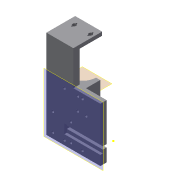
# Autodesk Inventor part: cellSTORM_inverted_Laser_10x_laserscanner_left_v2
Saved by Autodesk Inventor 2019.4 (Build 234330000, 330)
## iProperties
Created: 2020-11-05
Part Number: cellSTORM_inverted_Laser_10x_laserscanner_left_v2
Material: Generic
Document SubType Name: Modeling
Designer: diederichbenedict
Density: 1 g/cm^3
Appearance: Default
Author: diederichbenedict
Autodesk Inventor part; units mm, degrees
ref_plane "YZ Plane" through (0, 0, 0) normal (1, 0, 0) x (0, 1, 0)
ref_plane "Work Plane16" through (-37.5, 5.5, 41.5) normal (0, 0, -1) x (-1, 0, 0)
sketch "Sketch19" plane through (-37.5, 5.5, 41.5) normal (0, 0, -1) x (-1, 0, 0)
  circle A0 centre (-10, -25) radius 1.45 construction
  circle A1 centre (10, -25) radius 1.45 construction
  circle A2 centre (10, 25) radius 1.45 construction
  line L0 (-30, 28) -> (-30, -28) construction
  line L1 (28, 30) -> (-28, 30) construction
  line L2 (-30, -28) -> (-30, 28) construction
  line L3 (30, 28) -> (30, -28) construction
  line L4 (-28, -30) -> (28, -30) construction
  line L5 (-30, 0) -> (12.4264, 0) construction
  line L6 (0, 30) -> (30, 30)
  line L7 (30, 30) -> (30, 0)
  line L8 (30, 0) -> (41.9908, 0)
  line L9 (41.9908, -33.8566) -> (30, -30)
  line L10 (30, -30) -> (-30, -30)
  line L11 (-30, -30) -> (-30, 0)
  circle A3 centre (10, -25) radius 1.45
  circle A4 centre (10, 25) radius 1.45
  line L12 (0.5, 63.5) -> (25.5, 63.5)
  line L13 (0.5, 64.5) -> (25.5, 64.5)
  line L14 (30, 30) -> (0, 30)
  line L15 (0, 30) -> (0, 68.5)
  line L16 (0, 68.5) -> (30, 68.5)
  line L17 (30, 68.5) -> (30, 30)
  line L18 (0, 30) -> (-30, 30)
  line L19 (-30, 30) -> (-30, 0)
  circle A5 centre (-10, 25) radius 1.5209
  line L20 (30, 0.4817) -> (30, -30)
  circle A6 centre (-10, -25) radius 1.45
  point P0 (-37.5, -5.5)
  dimension "d106" = 4
  constraints: 42 end point, 8 horizontal, 7 centre point, 3 coincident, 3 concentric, 3 midpoint, 3 parallel, 3 vertical, 2 point on line, 1 collinear, 1 perpendicular, 18 other
  measures "d106" distance between parallel lines of L13 L16
extrude "Extrusion16" add sketch "Sketch19" along normal blind 7
ref_plane "Work Plane18" through (-80.5, 4.5, 11.5376) normal (0, 1, 0) x (0, 0, 1)
ref_plane "Work Plane19" through (-100.5, 11.5, 5.5) normal (0, 1, 0) x (0, 0, 1)
sketch "Sketch20" plane through (-79.4908, -24.5, 41.5) normal (0, 1, 0) x (1, 0, 0)
  line L0 (11.9908, 7) -> (41.9908, 7) projected
  line L1 (-5.0092, 36) -> (4.7181, 36)
  line L2 (4.7181, 36) -> (4.7181, 15.0376)
  line L3 (4.7181, 15.0376) -> (-5.0092, 15.0376)
  line L4 (21.7615, 7) -> (4.7181, 36)
  line L5 (21.7615, 7) -> (11.9908, 7)
  line L6 (-5.0092, 20.603) -> (-5.0092, 32.1376)
  line L7 (-5.0092, 36) -> (-5.0092, 15.0376)
  line L8 (-6.0092, 36) -> (-5.0092, 36)
  line L9 (-6.0092, 15.0376) -> (-5.0092, 15.0376)
  line L10 (4.7181, 15.0376) -> (11.9908, 15.0376)
  line L11 (11.9908, 15.0376) -> (11.9908, 7)
  point P0 (79.4908, 41.5)
  point P1 (28.1756, 7)
  dimension "d161" = 0
  dimension "d162" = 0
  constraints: 22 end point, 4 horizontal, 3 perpendicular, 1 collinear, 1 parallel, 1 point on line, 1 vertical, 6 other
  measures "d161" distance between parallel lines of L8 L1
  measures "d162" distance between parallel lines of L9 L3
extrude "Extrusion17" add sketch "Sketch20" along normal up to surface (36 mm away)
sketch "Sketch21" plane through (-84.5, -28.3595, 5.5) normal (-1, 0, 0) x (0, 0, 1)
  circle A0 centre (17.7, 9.3595) radius 1
  circle A1 centre (2.2, 30.8595) radius 1
  circle A2 centre (22.7, 37.3595) radius 1
  circle A3 centre (12.7, 19.8595) radius 2.6486
  line L0 (6.3352, 35.6445) -> (19.7051, 35.6445)
  line L1 (19.7051, 35.6445) -> (19.7051, 12.3611)
  line L2 (19.7051, 12.3611) -> (6.3352, 12.3611)
  line L3 (6.3352, 12.3611) -> (6.3352, 35.6445)
  line L4 (6.3352, 35.6445) -> (19.7051, 12.3611) construction
  line L5 (19.7051, 35.6445) -> (6.3352, 12.3611) construction
  circle A4 centre (17.7, 9.3595) radius 0.75
  circle A5 centre (2.2, 30.8595) radius 0.75
  circle A6 centre (22.7, 37.3595) radius 0.75
  point P0 (13.0201, 24.0028)
  dimension "d154" = 1.5
  dimension "d155" = 1.5
  dimension "d156" = 1.5
  constraints: 12 end point, 7 centre point, 3 coincident, 2 midpoint, 2 parallel, 1 horizontal, 1 perpendicular, 8 other
  measures "d154" diameter of A4
  measures "d155" diameter of A5
  measures "d156" diameter of A6
extrude "Extrusion18" cut sketch "Sketch21" against normal through all contours A3 | L0 L1 L2 L3 | A4 | A5 | A6
sketch "Sketch23" plane through (-37.5, 5.5, 34.5) normal (0, 0, -1) x (-1, 0, 0)
  line L0 (30, 6) -> (30, 68.5) projected
  line L1 (30, 68.5) -> (0, 68.5) projected
  line L2 (0, 68.5) -> (0, 30) projected
  line L3 (-30, 30) -> (-30, -30) projected
  line L4 (-30, -30) -> (20.2293, -30) projected
  circle A0 centre (10, -25) radius 1.45 projected
  circle A1 centre (10, 25) radius 1.45 projected
  line L5 (30, 68.5) -> (0, 68.5) projected
  line L6 (0.5, 64.5) -> (25.5, 64.5)
  line L7 (30, 68.5) -> (0, 68.5)
  line L8 (0, 68.5) -> (0, 64.5)
  line L9 (0, 64.5) -> (30, 64.5)
  line L10 (30, 64.5) -> (30, 68.5)
  line L11 (0, 30) -> (-30, 30) projected
  line L12 (20.2293, 6) -> (30, 6) projected
  line L13 (20.2293, -30) -> (20.2293, 6) projected
  point P0 (-37.5, -5.5)
  constraints: 10 end point, 2 horizontal, 2 parallel, 1 perpendicular, 1 point on line, 2 other
extrude "Extrusion20" add sketch "Sketch23" along normal blind 25 contours L9 L6 L2 L1 L0
sketch "Sketch24" plane through (-67.5, 74, 41.5) normal (0, 1, 0) x (1, 0, 0)
  circle A0 centre (6.5, 16.125) radius 1
  arc A1 (26, 21) -> (26, 25) centre (26, 23) ccw
  arc A2 (8, 25) -> (8, 21) centre (8, 23) ccw
  point P0 (67.5, 41.5)
  constraints: 4 point on circle, 3 centre point, 10 other
hole "Hole4" at (-59.5, 74, 18.5) at (-41.5, 74, 18.5) direction (0, -1, 0) diameter 4 depth 20 tip angle 118
sketch "Sketch25" plane through (-7.5, -24.5, 41.5) normal (1, 0, 0) x (0, 0, -1)
  line L0 (8, 17.4) -> (13.6, 17.4)
  line L1 (8, 14.6) -> (13.6, 14.6)
  line L2 (0, 0) -> (0, 98.5) projected
  line L3 (0, 21.0329) -> (2.8171, 21.0329)
  line L4 (2.8171, 21.0329) -> (2.8171, 10.7174)
  line L5 (2.8171, 10.7174) -> (0, 10.7174)
  line L6 (0, 10.7174) -> (0, 21.0329)
  line L7 (0.911, 17.6) -> (8.1191, 17.6)
  line L8 (8.1191, 17.6) -> (8.1191, 14.4)
  line L9 (8.1191, 14.4) -> (0.911, 14.4)
  line L10 (0.911, 14.4) -> (0.911, 17.6)
  line L11 (0.911, 17.6) -> (8.1191, 14.4) construction
  line L12 (8.1191, 17.6) -> (0.911, 14.4) construction
  circle A0 centre (23, 16) radius 2.5
  point P0 (41.5, 24.5)
  point P1 (4.5151, 16)
  dimension "d116" = 3.2
  dimension "d117" = 0
  constraints: 24 end point, 4 horizontal, 4 parallel, 2 midpoint, 2 perpendicular, 1 centre point, 1 point on line, 6 other
  measures "d116" distance of L7.end L8.end
  measures "d117" vertical distance of point (4.515, 16) A0.centre
extrude "Extrusion21" cut sketch "Sketch25" against normal blind 40 contours L2 L3 L4 L7 L10 L9 L5 | L9 L10 L7 L4 | L4 L7 L8 L9
ref_plane "Work Plane17" through (-65.74, 21.754, 18.5) normal (0, 1, 0) x (1, 0, 0)
sketch "Sketch26" plane through (-65.74, 21.754, 18.5) normal (0, 1, 0) x (1, 0, 0)
  circle A0 centre (15.24, 0) radius 15.24
  circle A1 centre (15.24, 0) radius 15.44
  line L0 (30.6779, -0.2548) -> (35.3241, -0.2548)
  line L1 (35.3241, -0.2548) -> (35.3241, -16)
  line L2 (58.24, -16) -> (8.0107, -16) projected
  line L3 (1.3147, -16) -> (35.3241, -16)
  arc A2 (-0.1726, -0.9196) -> (30.6779, -0.2548) centre (15.24, 0) ccw
  line L4 (-1.76, -16) -> (-1.76, -0.2548)
  line L5 (-1.76, -0.2548) -> (-0.1979, -0.2548)
  line L6 (-1.76, -16) -> (28.24, -16) projected
  line L7 (-1.76, -16) -> (28.24, -16)
  point P0 (65.74, 18.5)
  point P1 (14.4247, -16)
  dimension "d120" = 0.2
  constraints: 12 end point, 5 point on circle, 3 centre point, 3 horizontal, 2 concentric, 2 perpendicular, 1 point on line, 1 vertical, 2 other
  measures "d120" radial gap between concentric circles of A0 A1
extrude "Extrusion22" add sketch "Sketch26" along normal up to surface (24 mm away) from surface at -10.254 contours A1 L0 L1 L2 L3 L6 L4 L5
sketch "Sketch27" plane through (-30.4159, 35.5, 18.7548) normal (0, 0, -1) x (1, 0, 0)
  line L0 (-4.6462, 0) -> (0, 0) projected
  line L1 (-4.6462, 24) -> (-4.6462, 0) projected
  line L2 (0, 24) -> (0, 0) projected
  line L3 (-4.6462, 24) -> (0, 24) projected
  point P0 (30.4159, 35.5)
  point P1 (-2.3667, 19.6692)
  point P2 (-2.1061, 5.0728)
  point P3 (-54.438, 29.3311)
  point P4 (-55.6864, 54.2345)
  point P5 (7.1017, 19.6692)
hole "Hole5" at (-32.7825, 15.8308, 18.7548) at (-32.522, 30.4272, 18.7548) at (-86.1023, -18.7345, 18.7548) at (-84.8539, 6.1689, 18.7548) at (-23.3142, 15.8308, 18.7548) direction (0, 0, 1) diameter 2.9 end through all both
sketch "Sketch28" plane through (-37.5, 5.5, 34.5) normal (0, 0, -1) x (-1, 0, 0)
  point P0 (-37.5, -5.5)
sketch "Sketch29" plane through (-37.5, 5.5, 34.5) normal (0, 0, -1) x (-1, 0, 0)
  circle A0 centre (10, -25) radius 1.45 projected
  line L0 (-30, 30) -> (-30, -12.4) projected
  line L1 (-30, -12.4) -> (10, -12.4) projected
  line L2 (10, -12.4) -> (10, -15.6) projected
  line L3 (10, -15.6) -> (-30, -15.6) projected
  line L4 (-30, -15.6) -> (-30, -30) projected
  line L5 (-30, -30) -> (20.2293, -30) projected
  line L6 (12, -13) -> (13, -14)
  line L7 (4.9159, -8.7443) -> (17.0576, -20.886)
  line L8 (17.0576, -20.886) -> (14.9363, -23.0073)
  line L9 (14.9363, -23.0073) -> (2.7946, -10.8656)
  line L10 (2.7946, -10.8656) -> (4.9159, -8.7443)
  line L11 (6.3301, -7.3301) -> (18.4718, -19.4718)
  line L12 (18.4718, -19.4718) -> (20.5931, -17.3505)
  line L13 (20.5931, -17.3505) -> (8.4514, -5.2088)
  line L14 (8.4514, -5.2088) -> (6.3301, -7.3301)
  line L15 (30, 6) -> (30, 64.5) projected
  line L16 (30, 64.5) -> (0, 64.5) projected
  line L17 (0, 64.5) -> (0, 30) projected
  line L18 (0, 30) -> (-30, 30) projected
  line L19 (20.2293, -30) -> (20.2293, 6) projected
  line L20 (20.2293, 6) -> (30, 6) projected
  point P0 (-37.5, -5.5)
  dimension "d132" = 3
  dimension "d133" = 3
  dimension "d134" = 0
  dimension "d135" = 0
  dimension "d136" = 2
  dimension "d137" = 0
  constraints: 18 end point, 4 parallel, 2 perpendicular, 3 other
  measures "d132" distance between parallel lines of L7 L9
  measures "d133" distance between parallel lines of L13 L11
  measures "d134" distance between parallel lines of L14 L10
  measures "d135" distance between parallel lines of L12 L8
  measures "d136" distance between parallel lines of L11 L7
  measures "d137" distance between parallel lines of L11 L6
extrude "Extrusion23" add sketch "Sketch29" along normal blind 10 contours L9 L10 L7 L1 | L1 L7 L2 L3 L9 | L3 L2 L7 L8 L9 | L19 L12 L11 L6 L14 L13 | L13 L12 L19
sketch "Sketch30" plane through (-52.4363, -17.5073, 34.5) normal (0.7071068, -0.7071068, 0) x (-0.7071068, -0.7071068, 0)
  line L0 (0, 0) -> (-10.4755, 0) projected
  line L1 (0, 0) -> (0, 10) projected
  line L2 (-17.1709, 10) -> (0, 10) projected
  line L3 (-17.1709, 0) -> (-17.1709, 10) projected
  line L4 (-15.001, 0) -> (-17.1709, 0) projected
  line L5 (-10.4755, 0) -> (-15.001, 0) projected
  ellipse E0 centre (-38.851, 16) end of major axis (-38.851, 0.56) minor radius 10.9177 (-49.7672, 15.7452) -> (-27.9347, 15.7452) ccw projected
  circle A0 centre (-29.7987, 7.3684) radius 1.45
  circle A1 centre (-13.6778, 7.3684) radius 1.45
  circle A2 centre (-3.6035, 7.3684) radius 1.45
  point P0 (-49.4576, 34.5)
  point P1 (-6.7215, 15.7452)
  point P2 (-28.554, 15.7452)
  dimension "d140" = 2.9
  dimension "d152" = 2.9
  dimension "d153" = 2.9
  constraints: 3 centre point, 2 other
  measures "d140" diameter of A0
  measures "d152" diameter of A1
  measures "d153" diameter of A2
extrude "Extrusion24" cut sketch "Sketch30" against normal blind 10 contours A0 E0 | E0 A0 | A1 | A2
sketch "Sketch31" plane through (-37.5, 5.5, 34.5) normal (0, 0, -1) x (-1, 0, 0)
  line L0 (14.9363, -23.0073) -> (7.5289, -15.6) projected
  line L1 (7.5289, -15.6) -> (-30, -15.6) projected
  line L2 (-30, -15.6) -> (-30, -30) projected
  line L3 (-30, -30) -> (20.2293, -30) projected
  line L4 (-30, 30) -> (-30, -12.4) projected
  line L5 (-30, -12.4) -> (4.3289, -12.4) projected
  line L6 (4.3289, -12.4) -> (2.7946, -10.8656) projected
  line L7 (2.7946, -10.8656) -> (4.9159, -8.7443) projected
  line L8 (4.9159, -8.7443) -> (8.5716, -12.4) projected
  line L9 (8.5716, -12.4) -> (10, -12.4) projected
  line L10 (10, -12.4) -> (10, -13.8284) projected
  line L11 (10, -13.8284) -> (17.0576, -20.886) projected
  line L12 (6.3301, -7.3301) -> (8.4514, -5.2088) projected
  line L13 (8.4514, -5.2088) -> (20.2293, -16.9867) projected
  line L14 (18.4718, -19.4718) -> (6.3301, -7.3301) projected
  circle A0 centre (10, -25) radius 1.45 projected
  line L15 (22.8284, -23.8284) -> (2.8284, -23.8284)
  line L16 (2.8284, -23.8284) -> (2.8284, -3.8284)
  line L17 (2.8284, -3.8284) -> (22.8284, -3.8284)
  line L18 (22.8284, -3.8284) -> (22.8284, -23.8284)
  line L19 (13.4263, -14.4263) -> (11.3756, -12.3756) projected
  line L20 (22.8284, -23.8284) -> (2.8284, -3.8284) construction
  line L21 (2.8284, -23.8284) -> (22.8284, -3.8284) construction
  line L22 (30, 30) -> (30, 64.5) projected
  line L23 (30, 64.5) -> (0, 64.5) projected
  line L24 (0, 64.5) -> (0, 30) projected
  line L25 (-7.0841, 30) -> (-30, 30) projected
  line L26 (17.0576, -20.886) -> (14.9363, -23.0073) projected
  line L27 (20.2293, -17.7142) -> (18.4718, -19.4718) projected
  line L28 (20.2293, -16.9867) -> (20.2293, 6) projected
  line L29 (20.2293, -30) -> (20.2293, -17.7142) projected
  line L30 (0, 30) -> (30, 30) projected
  line L31 (20.2293, 6) -> (-7.0841, 6) projected
  line L32 (-7.0841, 6) -> (-7.0841, 30) projected
  point P0 (-37.5, -5.5)
  point P1 (12.8284, -13.8284)
  dimension "d143" = 20
  dimension "d144" = 20
  constraints: 12 end point, 2 midpoint, 2 parallel, 1 horizontal, 1 perpendicular, 1 point on line
  measures "d143" distance of L16.end L17.end
  measures "d144" distance of L15.end L16.end
hole "Hole6" at (-40.3284, 1.6716, 34.5) at (-60.3284, 1.6716, 34.5) at (-60.3284, -18.3284, 34.5) at (-40.3284, -18.3284, 34.5) direction (0, 0, 1) diameter 2.9 depth 20 tip angle 118
sketch "Sketch32" plane through (-99.5, 11.5, 5.8) normal (0, 1, 0) x (1, 0, 0)
  arc A0 (33.7368, -15.0302) -> (39.5379, -24.901) centre (49, -12.7) ccw projected
  line L0 (24.7272, 0.3) -> (32.5172, -12.9548) projected
  line L1 (32, -20.6624) -> (32, -12.9548) projected
  line L2 (32, -12.9548) -> (32.5172, -12.9548) projected
  circle A1 centre (49, -12.7) radius 15.44
  line L3 (15, 0.3) -> (24.7272, 0.3) projected
  line L4 (15, -20.6624) -> (15, 0.3) projected
  line L5 (32, -20.6624) -> (15, -20.6624) projected
  line L6 (33.7368, -15.0302) -> (39.5379, -24.901) projected
  point P0 (99.5, 5.8)
  constraints: 1 centre point, 1 coincident, 1 concentric
extrude "Extrusion25" cut sketch "Sketch32" against normal up to surface (11.2088 mm away) contours L6 A0 | A1 L6
sketch "Sketch33" plane through (-67.5, 74, 41.5) normal (0, 1, 0) x (1, 0, 0)
  circle A0 centre (8, 23) radius 2 projected
  circle A1 centre (26, 23) radius 2 projected
  line L0 (0, 0) -> (30, 0) projected
  line L1 (30, 0) -> (30, 32) projected
  line L2 (0, 32) -> (30, 32) projected
  line L3 (0, 0) -> (0, 32) projected
  line L4 (8, 20.538) -> (8, 25.462) construction
  line L5 (8.75, 20.538) -> (8.75, 25.462)
  line L6 (7.25, 25.462) -> (7.25, 20.538)
  arc A2 (7.25, 20.538) -> (8.75, 20.538) centre (8, 20.538) ccw
  arc A3 (8.75, 25.462) -> (7.25, 25.462) centre (8, 25.462) ccw
  line L7 (26, 20.538) -> (26, 25.462) construction
  line L8 (26.75, 20.538) -> (26.75, 25.462)
  line L9 (25.25, 25.462) -> (25.25, 20.538)
  arc A4 (25.25, 20.538) -> (26.75, 20.538) centre (26, 20.538) ccw
  arc A5 (26.75, 25.462) -> (25.25, 25.462) centre (26, 25.462) ccw
  point P0 (67.5, 41.5)
  constraints: 16 end point, 8 point on circle, 8 tangent, 4 centre point, 3 parallel, 2 midpoint, 1 vertical
extrude "Extrusion26" cut sketch "Sketch33" against normal blind 10 contours L5 A0 L6 | A0 L6 A3 L5 | L5 A2 L6 A0 | L8 A1 L9 | A1 L9 A5 L8 | L8 A4 L9 A1
sketch "Sketch34" plane through (-67.5, -24.5, 41.5) normal (0, -1, 0) x (1, 0, 0)
  line L0 (60, 0) -> (0, 0) projected
  line L1 (0, 0) -> (0, -15.0376) projected
  line L2 (-17, -15.0376) -> (0, -15.0376) projected
  line L3 (-17, -36) -> (-17, -15.0376) projected
  line L4 (-7.2728, -36) -> (-17, -36) projected
  line L5 (9.7707, -7) -> (-7.2728, -36) projected
  line L6 (60, -7) -> (9.7707, -7) projected
  line L7 (60, 0) -> (60, -7) projected
  line L8 (-7.2728, -36) -> (-17, -36) projected
  line L9 (-7.2728, -36) -> (20.9788, -36)
  line L10 (20.9788, -36) -> (20.9788, -7)
  point P0 (67.5, -41.5)
  constraints: 4 end point, 1 horizontal, 1 perpendicular, 1 point on line
extrude "Extrusion27" add sketch "Sketch34" against normal blind 3 contours L10 L9 L5 L6
sketch "Sketch35" plane through (-84.5, -24.5, 5.5) normal (-1, 0, 0) x (0, 0, 1)
  line L0 (-7.015, -5.6746) -> (29.4302, -5.6746)
  line L1 (29.4302, -5.6746) -> (29.4302, 44.1535)
  line L2 (29.4302, 44.1535) -> (-7.015, 44.1535)
  line L3 (-7.015, 44.1535) -> (-7.015, -5.6746)
  point P0 (-5.5, 24.5)
  constraints: 8 end point, 2 parallel, 1 horizontal, 1 perpendicular
extrude "Extrusion28" cut sketch "Sketch35" against normal blind 7
body "Solid3"
